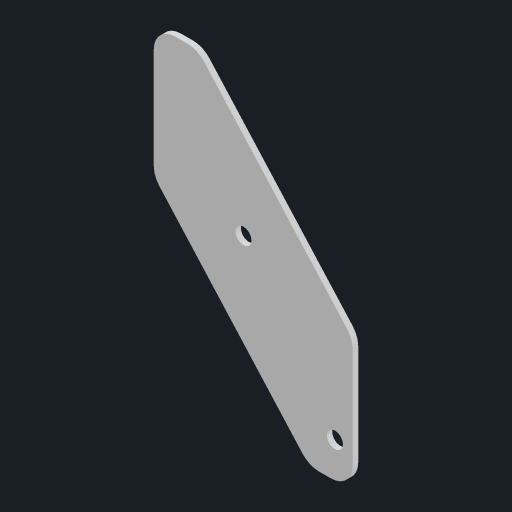
# Autodesk Inventor part: 6inSleds
Saved by Autodesk Inventor 2024.2 (Build 282272000, 272)
## iProperties
Created: 2024-01-29
Part Number: 6inSleds
Material: Generic
Document SubType Name: Sheet Metal
Designer: reima
Density: 1 g/cm^3
Sheet Metal Rule: Default
Appearance: Default
Author: reima
Autodesk Inventor part; units mm, degrees
ref_plane "YZ Plane" through (0, 0, 0) normal (1, 0, 0) x (0, 1, 0)
ref_plane "XZ Plane" through (0, 0, 0) normal (0, 1, 0) x (-1, 0, 0)
ref_plane "XY Plane" through (0, 0, 0) normal (0, 0, 1) x (1, 0, 0)
sketch "Sketch1" plane through (0, 0, 0) normal (0, 0, 1) x (1, 0, 0)
  circle A0 centre (-6.35, -152.4) radius 2.1844 construction
  circle A1 centre (-6.35, -139.7) radius 2.1844 construction
  circle A2 centre (6.35, -139.7) radius 2.1844 construction
  circle A3 centre (6.35, -152.4) radius 2.1844 construction
  circle A4 centre (0, -146.05) radius 2.1844 construction
  circle A5 centre (-6.35, -114.3) radius 2.1844 construction
  circle A6 centre (-6.35, -114.3) radius 34.925 construction
  line L0 (-41.275, -114.3) -> (60.325, -114.3) construction
  circle A7 centre (-6.35, -152.4) radius 9.525 construction
  line L1 (-30.7646, -139.3912) -> (10.8068, -185.8694)
  line L2 (-32.3816, -135.1578) -> (-32.3816, -105.8333)
  line L3 (-32.3816, -137.5833) -> (-3.057, -137.5833) construction
  line L4 (25.4, -152.3115) -> (25.4, -181.636)
  circle A8 centre (0, -146.05) radius 2.1844
  line L5 (15.5398, -187.986) -> (19.05, -187.986)
  line L6 (-26.0316, -99.4833) -> (-22.5214, -99.4833)
  line L7 (-17.7884, -101.6) -> (23.783, -148.0782)
  arc A9 (19.05, -187.986) -> (25.4, -181.636) centre (19.05, -181.636) ccw
  arc A10 (25.4, -152.3115) -> (23.783, -148.0782) centre (19.05, -152.3115) ccw
  arc A11 (-17.7884, -101.6) -> (-22.5214, -99.4833) centre (-22.5214, -105.8333) ccw
  arc A12 (-26.0316, -99.4833) -> (-32.3816, -105.8333) centre (-26.0316, -105.8333) ccw
  arc A13 (-32.3816, -135.1578) -> (-30.7646, -139.3912) centre (-26.0316, -135.1578) ccw
  arc A14 (10.8068, -185.8694) -> (15.5398, -187.986) centre (15.5398, -181.636) ccw
  circle A15 centre (20.2184, -152.3115) radius 2.3368 construction
  circle A16 centre (20.2184, -177.7115) radius 2.3495
  circle A17 centre (-6.35, -139.7) radius 2.3495
  point P0 (0, 0)
  point P1 (12.7, -158.75)
  point P2 (12.7, -187.986)
  point P3 (-32.3816, -99.4833)
  point P4 (25.4, -149.886)
  point P5 (25.4, -187.986)
  point P6 (-19.6816, -99.4833)
extrude "Plate1" add sketch "Sketch1" along normal blind 1.5875 contours A13 L2 A12 L6 A11 L7 A10 L4 A9 L5 A14 L1 | A8
equation "\"d24\" = Thickness"
equation "\"BendRadius\" = Thickness"
equation "\"BendReliefWidth\" = Thickness"
equation "\"BendReliefDepth\" = 0.5 * Thickness"
equation "\"CornerReliefSize\" = 4 * Thickness"
equation "\"MinimumRemnant\" = 2 * Thickness"
equation "\"TransitionRadius\" = BendRadius"
equation "\"JacobiRadiusSize\" = BendRadius"
equation "\"GapSize\" = Thickness"
equation "\"Thickness\" = 1.5875"
body "Solid1"
